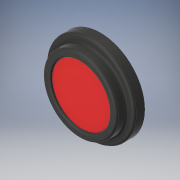
# Autodesk Inventor part: inkpad
Saved by Autodesk Inventor 2019 (Build 230136000, 136)
## iProperties
Created: 2020-10-20
Part Number: inkpad
Material: 一般
Document SubType Name: Modeling
Designer: Masato
Density: 1 g/cm^3
Appearance: 既定
Author: Masato
## iProperties of the stored document inkpad_3D プリント.ipt
Created: 2020-10-20
Part Number: inkpad_3D プリント
Material: 一般
Document SubType Name: Modeling
Designer: Masato
Density: 1 g/cm^3
Appearance: 既定
Author: Masato
Autodesk Inventor part; units mm, degrees
ref_plane "YZ Plane" through (0, 0, 0) normal (1, 0, 0) x (0, 1, 0)
ref_plane "XZ Plane" through (0, 0, 0) normal (0, 1, 0) x (-1, 0, 0)
ref_plane "XY Plane" through (0, 0, 0) normal (0, 0, 1) x (1, 0, 0)
sketch "スケッチ1" plane through (0, 0, 0) normal (0, 0, 1) x (1, 0, 0)
  circle A0 centre (0, 0) radius 21
  dimension "d0" = 42
  constraints: 1 centre point, 1 coincident
  measures "d0" diameter of A0
extrude "押し出し1" add sketch "スケッチ1" along normal blind 5
sketch "スケッチ2" plane through (0, 0, 5) normal (0, 0, 1) x (1, 0, 0)
  circle A0 centre (0, 0) radius 14
  circle A1 centre (0, 0) radius 17.5
  circle A2 centre (0, 0) radius 21 projected
  dimension "d3" = 28
  dimension "d8" = 7
  dimension "d9" = 3.5
  constraints: 2 centre point, 2 coincident
  measures "d3" diameter of A0
  measures "d8" radial gap between concentric circles of A2 A0
  measures "d9" radial gap between concentric circles of A0 A1
extrude "押し出し2" add sketch "スケッチ2" along normal blind 4 contours A0
extrude "押し出し3" add sketch "スケッチ2" along normal blind 5 contours A1
fillet "フィレット1" radius 1 4 edges at (-14, 0, 10) (-17.5, 0, 10) (-17.5, 0, 5) (-21, 0, 5)
equation "\"d9\" = 0.5 * d8"
